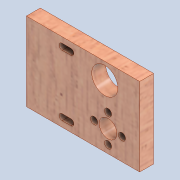
# Autodesk Inventor part: 0005-10-003 Actionare seringa
Saved by Autodesk Inventor 2020 (Build 240168000, 168)
## iProperties
Created: 2020-12-18
Part Number: 0005-10-003 Actionare seringa
Material: Wood (Maple)
Document SubType Name: Modeling
Designer: Iulian Bors
Density: 0.67 g/cm^3
Appearance: White Oak - Natural Medium Gloss
Mass: 13.719 g
Surface Area: 82.6049 cm^2
Volume: 20.4762 cm^3
Author: Iulian Bors
Subject: 003
Autodesk Inventor part; units mm, degrees
ref_plane "YZ Plane" through (0, 0, 0) normal (1, 0, 0) x (0, 1, 0)
ref_plane "XZ Plane" through (0, 0, 0) normal (0, 1, 0) x (-1, 0, 0)
ref_plane "XY Plane" through (0, 0, 0) normal (0, 0, 1) x (1, 0, 0)
sketch "Sketch1" plane through (0, 0, 0) normal (0, 0, 1) x (1, 0, 0)
  line L0 (-32.5, 22.5) -> (32.5, 22.5)
  line L1 (32.5, 22.5) -> (32.5, -22.5)
  line L2 (32.5, -22.5) -> (-32.5, -22.5)
  line L3 (-32.5, -22.5) -> (-32.5, 22.5)
  point P0 (0, 0)
  point P1 (0, 22.5)
  point P2 (-32.5, 0)
  dimension "d0" = 65
  dimension "d1" = 45
  constraints: 8 end point, 2 midpoint, 2 parallel, 1 horizontal, 1 horizontal alignment, 1 perpendicular, 1 vertical alignment
  measures "d0" distance of L0.start L0.end
  measures "d1" distance of L2.end L0.start
extrude "Extrusion1" add sketch "Sketch1" along normal blind 8
sketch "Sketch3" plane through (0, 0, 8) normal (0, 0, 1) x (1, 0, 0)
  line L0 (-32.5, -22.5) -> (32.5, -22.5) projected
  line L1 (32.5, -22.5) -> (32.5, 22.5) projected
  line L2 (32.5, 22.5) -> (-32.5, 22.5) projected
  line L3 (-32.5, 22.5) -> (-32.5, -22.5) projected
  line L4 (-12, 17.5) -> (-7, 17.5) construction
  line L5 (-12, 15.75) -> (-7, 15.75)
  line L6 (-7, 19.25) -> (-12, 19.25)
  arc A0 (-12, 19.25) -> (-12, 15.75) centre (-12, 17.5) ccw
  arc A1 (-7, 15.75) -> (-7, 19.25) centre (-7, 17.5) ccw
  line L7 (-12, -17.5) -> (-7, -17.5) construction
  line L8 (-12, -19.25) -> (-7, -19.25)
  line L9 (-7, -15.75) -> (-12, -15.75)
  arc A2 (-12, -15.75) -> (-12, -19.25) centre (-12, -17.5) ccw
  arc A3 (-7, -19.25) -> (-7, -15.75) centre (-7, -17.5) ccw
  circle A4 centre (-9.5, -17.5) radius 1.75 projected
  point P0 (0, 0)
  point P1 (-9.5, 17.5)
  point P2 (-9.5, -17.5)
  dimension "d8" = 5
  dimension "d9" = 3.5
  dimension "d10" = 5
  dimension "d16" = 5
  dimension "d17" = 23
  dimension "d18" = 5
  dimension "d36" = 23
  constraints: 16 end point, 8 point on circle, 8 tangent, 4 centre point, 3 parallel, 2 midpoint, 1 equal radius, 1 horizontal, 1 vertical alignment
  measures "d8" distance of L4.start L4.end
  measures "d9" diameter of A1
  measures "d10" distance of L7.start L7.end
  measures "d16" distance from line of L2 point (-9.5, 17.5)
  measures "d17" distance from line of point (-9.5, 17.5) L3
  measures "d18" distance between parallel lines of L0 L7
  measures "d36" distance from line of L3 A4.centre
extrude "Extrusion3" cut sketch "Sketch3" against normal through all contours A0 L6 A1 L5 | A2 L9 A4 L8 | A4 L9 A3 L8 | A4
sketch "Sketch4" plane through (0, 0, 8) normal (0, 0, 1) x (1, 0, 0)
  circle A0 centre (14.3605, -10) radius 11
  circle A1 centre (6.3605, -10) radius 2.05
  circle A2 centre (14.3605, -2) radius 2.05
  circle A3 centre (22.3605, -10) radius 2.05
  circle A4 centre (14.3605, -18) radius 2.05
  circle A5 centre (14.3605, -10) radius 5.1
  line L0 (32.5, -22.5) -> (32.5, 22.5) projected
  line L1 (-32.5, -22.5) -> (32.5, -22.5) projected
  dimension "d19" = 8
  dimension "d20" = 10.2
  dimension "d21" = 4.1
  dimension "d22" = 4.1
  dimension "d23" = 4.1
  dimension "d24" = 4.1
  dimension "d25" = 22
  dimension "d26" = 18.1395
  dimension "d27" = 8
  dimension "d28" = 8
  dimension "d29" = 8
  dimension "d30" = 12.5
  constraints: 6 centre point, 2 horizontal alignment, 2 vertical alignment, 1 concentric
  measures "d19" distance of A5.centre A2.centre
  measures "d20" diameter of A5
  measures "d21" diameter of A2
  measures "d22" diameter of A3
  measures "d23" diameter of A4
  measures "d24" diameter of A1
  measures "d25" diameter of A0
  measures "d26" distance from line of A0.centre L0
  measures "d27" distance of A0.centre A1.centre
  measures "d28" distance of A0.centre A3.centre
  measures "d29" distance of A4.centre A0.centre
  measures "d30" distance from line of L1 A0.centre
extrude "Extrusion4" cut sketch "Sketch4" against normal through all contours A1 | A2 | A3 | A4 | A5
sketch "Sketch5" plane through (0, 0, 8) normal (0, 0, 1) x (1, 0, 0)
  circle A0 centre (12.5, 13) radius 7.5
  circle A1 centre (14.3605, -10) radius 5.1 projected
  line L0 (32.5, -22.5) -> (32.5, 22.5) projected
  point P0 (0, 0)
  dimension "d31" = 15
  dimension "d32" = 23
  dimension "d33" = 20
  constraints: 1 centre point
  measures "d31" diameter of A0
  measures "d32" vertical distance of A1.centre A0.centre
  measures "d33" distance from line of L0 A0.centre
extrude "Extrusion5" cut sketch "Sketch5" against normal blind 10 contours A0
equation "\"d18\" = d16"
body "Solid1"
